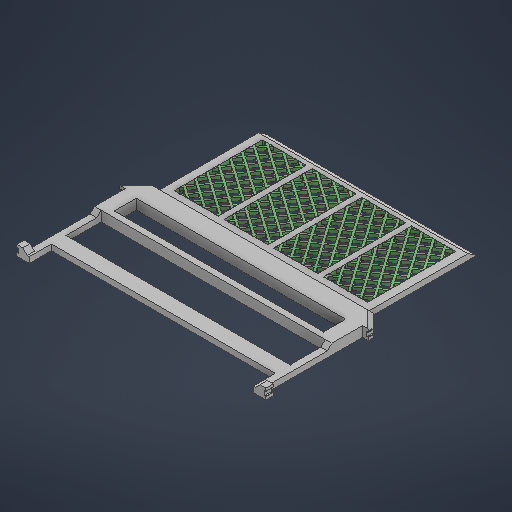
# Autodesk Inventor part: SACMI PH1500 FILLER BOX GRID-DRIVING
Saved by Autodesk Inventor 2025 (Build 290162000, 162)
## iProperties
Created: 2024-05-03
Part Number: SACMI PH1500 FILLER BOX GRID-DRIVING
Material: Generic
Document SubType Name: Modeling
Designer: zulet
Density: 1 g/cm^3
Appearance: Smooth - Medium Gray
Author: zulet
Autodesk Inventor part; units mm, degrees
(part 1 of 2)
ref_plane "YZ Plane" through (0, 0, 0) normal (1, 0, 0) x (0, 1, 0)
ref_plane "XZ Plane" through (0, 0, 0) normal (0, 1, 0) x (-1, 0, 0)
ref_plane "XY Plane" through (0, 0, 0) normal (0, 0, 1) x (1, 0, 0)
sketch "Sketch1" plane through (0, 0, 0) normal (0, 1, 0) x (-1, 0, 0)
  line L0 (-2029.8955, 1380.0763) -> (2005.9504, 1380.0763) construction
  line L1 (2005.9504, 1380.0763) -> (2005.9504, -2689.5627) construction
  line L2 (2005.9504, -2689.5627) -> (-2029.8955, -2689.5627) construction
  line L3 (-2029.8955, -2689.5627) -> (-2029.8955, 1380.0763) construction
  line L4 (810, 0) -> (765, 0)
  line L5 (715, -840) -> (745, -840)
  line L6 (745, -840) -> (850, -735)
  line L7 (850, -735) -> (850, -700)
  line L8 (850, -700) -> (810, -700)
  line L9 (810, -700) -> (810, 0)
  line L10 (715, -840) -> (715, -1515)
  line L11 (715, -1515) -> (0, -1515)
  line L12 (0, -1515) -> (0, -680)
  line L13 (0, -680) -> (715, -680)
  line L14 (765, -490) -> (0, -490)
  line L15 (0, -490) -> (0, -530)
  line L16 (0, -530) -> (715, -530)
  line L17 (715, -530) -> (715, -680)
  line L18 (765, -490) -> (765, -250)
  line L19 (765, -250) -> (0, -250)
  line L20 (0, -250) -> (0, -150)
  line L21 (0, -150) -> (765, -150)
  line L22 (765, -150) -> (765, 0)
  line L23 (810, 0) -> (850, 0)
  line L24 (850, 0) -> (850, -50)
  line L25 (850, -50) -> (810, -50)
  line L26 (810, -50) -> (810, 0)
  line L27 (0, 0) -> (0, -1515) construction
  line L28 (0, 0) -> (850, 0) construction
  line L29 (715, -840) -> (715, -680)
  line L30 (765, -490) -> (810, -490)
  line L31 (715, -840) -> (0, -840)
  point P0 (830, -50)
  point P1 (715, -605)
  point P2 (0, -840)
  dimension "d1" = 4035.8459
  dimension "d24" = 45
  dimension "d25" = 150
  dimension "d26" = 100
  dimension "d27" = 240
  dimension "d28" = 40
  dimension "d29" = 150
  dimension "d32" = 810
  dimension "d33" = 50
  dimension "d43" = 650
  dimension "d45" = 140
  dimension "d46" = 45
  dimension "d48" = 35
  dimension "d49" = 40
  dimension "d50" = 95
  dimension "d57" = 780
  constraints: 56 end point, 13 perpendicular, 7 horizontal, 6 collinear, 4 point on line, 3 vertical, 2 midpoint, 2 parallel, 2 other
  measures "d1" distance of L1.end L2.end
  measures "d24" distance between parallel lines of L22 L9
  measures "d25" distance between parallel lines of L4 L21
  measures "d26" distance between parallel lines of L19 L21
  measures "d27" distance between parallel lines of L14 L19
  measures "d28" distance between parallel lines of L16 L14
  measures "d29" distance between parallel lines of L13 L16
  measures "d32" distance between parallel lines of L27 L9
  measures "d33" distance of L23.end L24.end
  measures "d43" distance from line of point (830, -50) L8
  measures "d45" distance between parallel lines of L8 L5
  measures "d46" angle of L5 L6
  measures "d48" distance of L6.end L7.end
  measures "d49" distance between parallel lines of L9 L24
  measures "d50" distance from line of L9 point (715, -605)
  measures "d57" distance from line of L11 L6.end
extrude "Extrusion1" add sketch "Sketch1" along normal blind 70 contours L23 L24 L25 L9 | L9 L8 L7 L6 L5 L29 L17 L16 L15 L14 L30 | L31 L12 L13 L29
extrude "Extrusion3" add sketch "Sketch1" along normal blind 40 contours L9 L30 L18 L19 L20 L21 L22 L4 | L31 L12 L13 L29 | L10 L11 L12 L31
sketch "Sketch2" plane through (0, 40, 0) normal (0, 1, 0) x (1, 0, 0)
  line L0 (-660, 1485) -> (-360, 1485)
  line L1 (-360, 1485) -> (-360, 885)
  line L2 (-360, 885) -> (-660, 885)
  line L3 (-660, 885) -> (-660, 1485)
  line L4 (0, 1515) -> (-715, 1515) projected
  line L5 (-850, 735) -> (-850, 700) projected
  line L6 (-320, 885) -> (-20, 885)
  line L7 (-20, 885) -> (-20, 1485)
  line L8 (-20, 1485) -> (-320, 1485)
  line L9 (-320, 1485) -> (-320, 885)
  point P0 (0, 0)
  dimension "d58" = 300
  dimension "d59" = 600
  dimension "d60" = 30
  dimension "d61" = 190
  dimension "d62" = 300
  dimension "d63" = 600
  dimension "d64" = 40
  dimension "d65" = 30
  constraints: 16 end point, 4 parallel, 2 horizontal, 2 perpendicular
  measures "d58" distance of L1.end L2.end
  measures "d59" distance of L0.end L1.end
  measures "d60" distance between parallel lines of L4 L0
  measures "d61" distance between parallel lines of L3 L5
  measures "d62" distance of L8.end L7.end
  measures "d63" distance of L7.end L6.end
  measures "d64" distance between parallel lines of L1 L9
  measures "d65" distance between parallel lines of L4 L8
extrude "Extrusion4" cut sketch "Sketch2" against normal blind 40
sketch "Sketch3" plane through (0, 40, 0) normal (0, 1, 0) x (1, 0, 0)
  line L0 (273.75, 1258.6647) -> (232.7924, 1287.3435)
  line L1 (232.7924, 1287.3435) -> (261.4712, 1328.3011)
  line L2 (261.4712, 1328.3011) -> (302.4288, 1299.6223)
  line L3 (302.4288, 1299.6223) -> (273.75, 1258.6647)
  line L4 (-360, 885) -> (-660, 885) projected
  line L5 (220.5051, 1295.9471) -> (179.5475, 1324.626)
  line L6 (179.5475, 1324.626) -> (208.2263, 1365.5836)
  line L7 (208.2263, 1365.5836) -> (249.1839, 1336.9047)
  line L8 (249.1839, 1336.9047) -> (220.5051, 1295.9471)
  line L9 (167.2602, 1333.2296) -> (126.3026, 1361.9084)
  line L10 (126.3026, 1361.9084) -> (154.9815, 1402.866)
  line L11 (154.9815, 1402.866) -> (195.9391, 1374.1872)
  line L12 (195.9391, 1374.1872) -> (167.2602, 1333.2296)
  line L13 (114.0154, 1370.5121) -> (73.0577, 1399.1909)
  line L14 (73.0577, 1399.1909) -> (101.7366, 1440.1485)
  line L15 (101.7366, 1440.1485) -> (142.6942, 1411.4697)
  line L16 (142.6942, 1411.4697) -> (114.0154, 1370.5121)
  line L17 (60.7705, 1407.7945) -> (19.8129, 1436.4734)
  line L18 (19.8129, 1436.4734) -> (48.4917, 1477.431)
  line L19 (48.4917, 1477.431) -> (89.4493, 1448.7521)
  line L20 (89.4493, 1448.7521) -> (60.7705, 1407.7945)
  line L21 (7.5256, 1445.077) -> (-33.432, 1473.7558)
  line L22 (-33.432, 1473.7558) -> (-4.7532, 1514.7134)
  line L23 (-4.7532, 1514.7134) -> (36.2044, 1486.0346)
  line L24 (36.2044, 1486.0346) -> (7.5256, 1445.077)
  line L25 (-45.7193, 1482.3595) -> (-86.6769, 1511.0383)
  line L26 (-86.6769, 1511.0383) -> (-57.9981, 1551.9959)
  line L27 (-57.9981, 1551.9959) -> (-17.0405, 1523.3171)
  line L28 (-17.0405, 1523.3171) -> (-45.7193, 1482.3595)
  line L29 (-98.9642, 1519.6419) -> (-139.9218, 1548.3208)
  line L30 (-139.9218, 1548.3208) -> (-111.243, 1589.2784)
  line L31 (-111.243, 1589.2784) -> (-70.2854, 1560.5995)
  line L32 (-70.2854, 1560.5995) -> (-98.9642, 1519.6419)
  line L33 (-152.2091, 1556.9244) -> (-193.1667, 1585.6032)
  line L34 (-193.1667, 1585.6032) -> (-164.4878, 1626.5608)
  line L35 (-164.4878, 1626.5608) -> (-123.5302, 1597.882)
  line L36 (-123.5302, 1597.882) -> (-152.2091, 1556.9244)
  line L37 (-205.4539, 1594.2069) -> (-246.4115, 1622.8857)
  line L38 (-246.4115, 1622.8857) -> (-217.7327, 1663.8433)
  line L39 (-217.7327, 1663.8433) -> (-176.7751, 1635.1645)
  line L40 (-176.7751, 1635.1645) -> (-205.4539, 1594.2069)
  line L41 (-258.6988, 1631.4894) -> (-299.6564, 1660.1682)
  line L42 (-299.6564, 1660.1682) -> (-270.9776, 1701.1258)
  line L43 (-270.9776, 1701.1258) -> (-230.02, 1672.447)
  line L44 (-230.02, 1672.447) -> (-258.6988, 1631.4894)
  line L45 (-311.9437, 1668.7718) -> (-352.9013, 1697.4506)
  line L46 (-352.9013, 1697.4506) -> (-324.2225, 1738.4082)
  line L47 (-324.2225, 1738.4082) -> (-283.2649, 1709.7294)
  line L48 (-283.2649, 1709.7294) -> (-311.9437, 1668.7718)
  line L49 (-365.1886, 1706.0543) -> (-406.1462, 1734.7331)
  line L50 (-406.1462, 1734.7331) -> (-377.4674, 1775.6907)
  line L51 (-377.4674, 1775.6907) -> (-336.5098, 1747.0119)
  line L52 (-336.5098, 1747.0119) -> (-365.1886, 1706.0543)
  line L53 (-418.4335, 1743.3368) -> (-459.3911, 1772.0156)
  line L54 (-459.3911, 1772.0156) -> (-430.7123, 1812.9732)
  line L55 (-430.7123, 1812.9732) -> (-389.7547, 1784.2944)
  line L56 (-389.7547, 1784.2944) -> (-418.4335, 1743.3368)
  line L57 (-471.6784, 1780.6192) -> (-512.636, 1809.298)
  line L58 (-512.636, 1809.298) -> (-483.9571, 1850.2556)
  line L59 (-483.9571, 1850.2556) -> (-442.9995, 1821.5768)
  line L60 (-442.9995, 1821.5768) -> (-471.6784, 1780.6192)
  line L61 (236.4675, 1205.4198) -> (195.5099, 1234.0986)
  line L62 (195.5099, 1234.0986) -> (224.1888, 1275.0562)
  line L63 (224.1888, 1275.0562) -> (265.1464, 1246.3774)
  line L64 (265.1464, 1246.3774) -> (236.4675, 1205.4198)
  line L65 (183.2226, 1242.7023) -> (142.265, 1271.3811)
  line L66 (142.265, 1271.3811) -> (170.9439, 1312.3387)
  line L67 (170.9439, 1312.3387) -> (211.9015, 1283.6599)
  line L68 (211.9015, 1283.6599) -> (183.2226, 1242.7023)
  line L69 (129.9778, 1279.9847) -> (89.0202, 1308.6635)
  line L70 (89.0202, 1308.6635) -> (117.699, 1349.6211)
  line L71 (117.699, 1349.6211) -> (158.6566, 1320.9423)
  line L72 (158.6566, 1320.9423) -> (129.9778, 1279.9847)
  line L73 (76.7329, 1317.2672) -> (35.7753, 1345.946)
  line L74 (35.7753, 1345.946) -> (64.4541, 1386.9036)
  line L75 (64.4541, 1386.9036) -> (105.4117, 1358.2248)
  line L76 (105.4117, 1358.2248) -> (76.7329, 1317.2672)
  line L77 (23.488, 1354.5497) -> (-17.4696, 1383.2285)
  line L78 (-17.4696, 1383.2285) -> (11.2092, 1424.1861)
  line L79 (11.2092, 1424.1861) -> (52.1668, 1395.5073)
  line L80 (52.1668, 1395.5073) -> (23.488, 1354.5497)
  line L81 (-29.7569, 1391.8321) -> (-70.7145, 1420.5109)
  line L82 (-70.7145, 1420.5109) -> (-42.0357, 1461.4686)
  line L83 (-42.0357, 1461.4686) -> (-1.0781, 1432.7897)
  line L84 (-1.0781, 1432.7897) -> (-29.7569, 1391.8321)
  line L85 (-83.0018, 1429.1146) -> (-123.9594, 1457.7934)
  line L86 (-123.9594, 1457.7934) -> (-95.2805, 1498.751)
  line L87 (-95.2805, 1498.751) -> (-54.3229, 1470.0722)
  line L88 (-54.3229, 1470.0722) -> (-83.0018, 1429.1146)
  line L89 (-136.2466, 1466.3971) -> (-177.2043, 1495.0759)
  line L90 (-177.2043, 1495.0759) -> (-148.5254, 1536.0335)
  line L91 (-148.5254, 1536.0335) -> (-107.5678, 1507.3547)
  line L92 (-107.5678, 1507.3547) -> (-136.2466, 1466.3971)
  line L93 (-189.4915, 1503.6795) -> (-230.4491, 1532.3584)
  line L94 (-230.4491, 1532.3584) -> (-201.7703, 1573.316)
  line L95 (-201.7703, 1573.316) -> (-160.8127, 1544.6371)
  line L96 (-160.8127, 1544.6371) -> (-189.4915, 1503.6795)
  line L97 (-242.7364, 1540.962) -> (-283.694, 1569.6408)
  line L98 (-283.694, 1569.6408) -> (-255.0152, 1610.5984)
  line L99 (-255.0152, 1610.5984) -> (-214.0576, 1581.9196)
  line L100 (-214.0576, 1581.9196) -> (-242.7364, 1540.962)
  line L101 (-295.9813, 1578.2445) -> (-336.9389, 1606.9233)
  line L102 (-336.9389, 1606.9233) -> (-308.2601, 1647.8809)
  line L103 (-308.2601, 1647.8809) -> (-267.3025, 1619.2021)
  line L104 (-267.3025, 1619.2021) -> (-295.9813, 1578.2445)
  line L105 (-349.2262, 1615.5269) -> (-390.1838, 1644.2058)
  line L106 (-390.1838, 1644.2058) -> (-361.505, 1685.1634)
  line L107 (-361.505, 1685.1634) -> (-320.5474, 1656.4845)
  line L108 (-320.5474, 1656.4845) -> (-349.2262, 1615.5269)
  line L109 (-402.4711, 1652.8094) -> (-443.4287, 1681.4882)
  line L110 (-443.4287, 1681.4882) -> (-414.7498, 1722.4458)
  line L111 (-414.7498, 1722.4458) -> (-373.7922, 1693.767)
  line L112 (-373.7922, 1693.767) -> (-402.4711, 1652.8094)
  line L113 (-455.7159, 1690.0919) -> (-496.6735, 1718.7707)
  line L114 (-496.6735, 1718.7707) -> (-467.9947, 1759.7283)
  line L115 (-467.9947, 1759.7283) -> (-427.0371, 1731.0495)
  line L116 (-427.0371, 1731.0495) -> (-455.7159, 1690.0919)
  line L117 (-508.9608, 1727.3743) -> (-549.9184, 1756.0532)
  line L118 (-549.9184, 1756.0532) -> (-521.2396, 1797.0108)
  line L119 (-521.2396, 1797.0108) -> (-480.282, 1768.3319)
  line L120 (-480.282, 1768.3319) -> (-508.9608, 1727.3743)
  line L121 (199.1851, 1152.1749) -> (158.2275, 1180.8537)
  line L122 (158.2275, 1180.8537) -> (186.9063, 1221.8113)
  line L123 (186.9063, 1221.8113) -> (227.8639, 1193.1325)
  line L124 (227.8639, 1193.1325) -> (199.1851, 1152.1749)
  line L125 (145.9402, 1189.4574) -> (104.9826, 1218.1362)
  line L126 (104.9826, 1218.1362) -> (133.6614, 1259.0938)
  line L127 (133.6614, 1259.0938) -> (174.619, 1230.415)
  line L128 (174.619, 1230.415) -> (145.9402, 1189.4574)
  line L129 (92.6953, 1226.7398) -> (51.7377, 1255.4187)
  line L130 (51.7377, 1255.4187) -> (80.4165, 1296.3763)
  line L131 (80.4165, 1296.3763) -> (121.3741, 1267.6974)
  line L132 (121.3741, 1267.6974) -> (92.6953, 1226.7398)
  line L133 (39.4504, 1264.0223) -> (-1.5072, 1292.7011)
  line L134 (-1.5072, 1292.7011) -> (27.1716, 1333.6587)
  line L135 (27.1716, 1333.6587) -> (68.1292, 1304.9799)
  line L136 (68.1292, 1304.9799) -> (39.4504, 1264.0223)
  line L137 (-13.7945, 1301.3048) -> (-54.7521, 1329.9836)
  line L138 (-54.7521, 1329.9836) -> (-26.0732, 1370.9412)
  line L139 (-26.0732, 1370.9412) -> (14.8844, 1342.2624)
  line L140 (14.8844, 1342.2624) -> (-13.7945, 1301.3048)
  line L141 (-67.0394, 1338.5872) -> (-107.997, 1367.2661)
  line L142 (-107.997, 1367.2661) -> (-79.3181, 1408.2237)
  line L143 (-79.3181, 1408.2237) -> (-38.3605, 1379.5448)
  line L144 (-38.3605, 1379.5448) -> (-67.0394, 1338.5872)
  line L145 (-120.2842, 1375.8697) -> (-161.2418, 1404.5485)
  line L146 (-161.2418, 1404.5485) -> (-132.563, 1445.5061)
  line L147 (-132.563, 1445.5061) -> (-91.6054, 1416.8273)
  line L148 (-91.6054, 1416.8273) -> (-120.2842, 1375.8697)
  line L149 (-173.5291, 1413.1522) -> (-214.4867, 1441.831)
  line L150 (-214.4867, 1441.831) -> (-185.8079, 1482.7886)
  line L151 (-185.8079, 1482.7886) -> (-144.8503, 1454.1098)
  line L152 (-144.8503, 1454.1098) -> (-173.5291, 1413.1522)
  line L153 (-226.774, 1450.4346) -> (-267.7316, 1479.1135)
  line L154 (-267.7316, 1479.1135) -> (-239.0528, 1520.0711)
  line L155 (-239.0528, 1520.0711) -> (-198.0952, 1491.3923)
  line L156 (-198.0952, 1491.3923) -> (-226.774, 1450.4346)
  line L157 (-280.0189, 1487.7171) -> (-320.9765, 1516.3959)
  line L158 (-320.9765, 1516.3959) -> (-292.2977, 1557.3535)
  line L159 (-292.2977, 1557.3535) -> (-251.3401, 1528.6747)
  line L160 (-251.3401, 1528.6747) -> (-280.0189, 1487.7171)
  line L161 (-333.2638, 1524.9996) -> (-374.2214, 1553.6784)
  line L162 (-374.2214, 1553.6784) -> (-345.5425, 1594.636)
  line L163 (-345.5425, 1594.636) -> (-304.5849, 1565.9572)
  line L164 (-304.5849, 1565.9572) -> (-333.2638, 1524.9996)
  line L165 (-386.5086, 1562.2821) -> (-427.4663, 1590.9609)
  line L166 (-427.4663, 1590.9609) -> (-398.7874, 1631.9185)
  line L167 (-398.7874, 1631.9185) -> (-357.8298, 1603.2397)
  line L168 (-357.8298, 1603.2397) -> (-386.5086, 1562.2821)
  line L169 (-439.7535, 1599.5645) -> (-480.7111, 1628.2433)
  line L170 (-480.7111, 1628.2433) -> (-452.0323, 1669.2009)
  line L171 (-452.0323, 1669.2009) -> (-411.0747, 1640.5221)
  line L172 (-411.0747, 1640.5221) -> (-439.7535, 1599.5645)
  line L173 (-492.9984, 1636.847) -> (-533.956, 1665.5258)
  line L174 (-533.956, 1665.5258) -> (-505.2772, 1706.4834)
  line L175 (-505.2772, 1706.4834) -> (-464.3196, 1677.8046)
  line L176 (-464.3196, 1677.8046) -> (-492.9984, 1636.847)
  line L177 (-546.2433, 1674.1295) -> (-587.2009, 1702.8083)
  line L178 (-587.2009, 1702.8083) -> (-558.5221, 1743.7659)
  line L179 (-558.5221, 1743.7659) -> (-517.5645, 1715.0871)
  line L180 (-517.5645, 1715.0871) -> (-546.2433, 1674.1295)
  line L181 (161.9026, 1098.93) -> (120.945, 1127.6088)
  line L182 (120.945, 1127.6088) -> (149.6238, 1168.5664)
  line L183 (149.6238, 1168.5664) -> (190.5814, 1139.8876)
  line L184 (190.5814, 1139.8876) -> (161.9026, 1098.93)
  line L185 (108.6577, 1136.2125) -> (67.7001, 1164.8913)
  line L186 (67.7001, 1164.8913) -> (96.3789, 1205.8489)
  line L187 (96.3789, 1205.8489) -> (137.3365, 1177.1701)
  line L188 (137.3365, 1177.1701) -> (108.6577, 1136.2125)
  line L189 (55.4128, 1173.495) -> (14.4552, 1202.1738)
  line L190 (14.4552, 1202.1738) -> (43.134, 1243.1314)
  line L191 (43.134, 1243.1314) -> (84.0917, 1214.4526)
  line L192 (84.0917, 1214.4526) -> (55.4128, 1173.495)
  line L193 (2.1679, 1210.7774) -> (-38.7897, 1239.4562)
  line L194 (-38.7897, 1239.4562) -> (-10.1108, 1280.4138)
  line L195 (-10.1108, 1280.4138) -> (30.8468, 1251.735)
  line L196 (30.8468, 1251.735) -> (2.1679, 1210.7774)
  line L197 (-51.0769, 1248.0599) -> (-92.0345, 1276.7387)
  line L198 (-92.0345, 1276.7387) -> (-63.3557, 1317.6963)
  line L199 (-63.3557, 1317.6963) -> (-22.3981, 1289.0175)
  line L200 (-22.3981, 1289.0175) -> (-51.0769, 1248.0599)
  line L201 (-104.3218, 1285.3424) -> (-145.2794, 1314.0212)
  line L202 (-145.2794, 1314.0212) -> (-116.6006, 1354.9788)
  line L203 (-116.6006, 1354.9788) -> (-75.643, 1326.3)
  line L204 (-75.643, 1326.3) -> (-104.3218, 1285.3424)
  line L205 (-157.5667, 1322.6248) -> (-198.5243, 1351.3037)
  line L206 (-198.5243, 1351.3037) -> (-169.8455, 1392.2613)
  line L207 (-169.8455, 1392.2613) -> (-128.8879, 1363.5824)
  line L208 (-128.8879, 1363.5824) -> (-157.5667, 1322.6248)
  line L209 (-210.8116, 1359.9073) -> (-251.7692, 1388.5861)
  line L210 (-251.7692, 1388.5861) -> (-223.0904, 1429.5437)
  line L211 (-223.0904, 1429.5437) -> (-182.1328, 1400.8649)
  line L212 (-182.1328, 1400.8649) -> (-210.8116, 1359.9073)
  line L213 (-264.0565, 1397.1898) -> (-305.0141, 1425.8686)
  line L214 (-305.0141, 1425.8686) -> (-276.3352, 1466.8262)
  line L215 (-276.3352, 1466.8262) -> (-235.3776, 1438.1474)
  line L216 (-235.3776, 1438.1474) -> (-264.0565, 1397.1898)
  line L217 (-317.3014, 1434.4722) -> (-358.259, 1463.1511)
  line L218 (-358.259, 1463.1511) -> (-329.5801, 1504.1087)
  line L219 (-329.5801, 1504.1087) -> (-288.6225, 1475.4298)
  line L220 (-288.6225, 1475.4298) -> (-317.3014, 1434.4722)
  line L221 (-370.5462, 1471.7547) -> (-411.5038, 1500.4335)
  line L222 (-411.5038, 1500.4335) -> (-382.825, 1541.3911)
  line L223 (-382.825, 1541.3911) -> (-341.8674, 1512.7123)
  line L224 (-341.8674, 1512.7123) -> (-370.5462, 1471.7547)
  line L225 (-423.7911, 1509.0372) -> (-464.7487, 1537.716)
  line L226 (-464.7487, 1537.716) -> (-436.0699, 1578.6736)
  line L227 (-436.0699, 1578.6736) -> (-395.1123, 1549.9948)
  line L228 (-395.1123, 1549.9948) -> (-423.7911, 1509.0372)
  line L229 (-477.036, 1546.3196) -> (-517.9936, 1574.9985)
  line L230 (-517.9936, 1574.9985) -> (-489.3148, 1615.9561)
  line L231 (-489.3148, 1615.9561) -> (-448.3572, 1587.2772)
  line L232 (-448.3572, 1587.2772) -> (-477.036, 1546.3196)
  line L233 (-530.2809, 1583.6021) -> (-571.2385, 1612.2809)
  line L234 (-571.2385, 1612.2809) -> (-542.5597, 1653.2385)
  line L235 (-542.5597, 1653.2385) -> (-501.6021, 1624.5597)
  line L236 (-501.6021, 1624.5597) -> (-530.2809, 1583.6021)
  line L237 (-583.5258, 1620.8846) -> (-624.4834, 1649.5634)
  line L238 (-624.4834, 1649.5634) -> (-595.8045, 1690.521)
  line L239 (-595.8045, 1690.521) -> (-554.8469, 1661.8422)
  line L240 (-554.8469, 1661.8422) -> (-583.5258, 1620.8846)
  line L241 (124.6201, 1045.6851) -> (83.6625, 1074.364)
  line L242 (83.6625, 1074.364) -> (112.3413, 1115.3216)
  line L243 (112.3413, 1115.3216) -> (153.2989, 1086.6427)
  line L244 (153.2989, 1086.6427) -> (124.6201, 1045.6851)
  line L245 (71.3752, 1082.9676) -> (30.4176, 1111.6464)
  line L246 (30.4176, 1111.6464) -> (59.0965, 1152.604)
  line L247 (59.0965, 1152.604) -> (100.0541, 1123.9252)
  line L248 (100.0541, 1123.9252) -> (71.3752, 1082.9676)
  line L249 (18.1304, 1120.2501) -> (-22.8272, 1148.9289)
  line L250 (-22.8272, 1148.9289) -> (5.8516, 1189.8865)
  line L251 (5.8516, 1189.8865) -> (46.8092, 1161.2077)
  line L252 (46.8092, 1161.2077) -> (18.1304, 1120.2501)
  line L253 (-35.1145, 1157.5325) -> (-76.0721, 1186.2114)
  line L254 (-76.0721, 1186.2114) -> (-47.3933, 1227.169)
  line L255 (-47.3933, 1227.169) -> (-6.4357, 1198.4901)
  line L256 (-6.4357, 1198.4901) -> (-35.1145, 1157.5325)
  line L257 (-88.3594, 1194.815) -> (-129.317, 1223.4938)
  line L258 (-129.317, 1223.4938) -> (-100.6382, 1264.4514)
  line L259 (-100.6382, 1264.4514) -> (-59.6806, 1235.7726)
  line L260 (-59.6806, 1235.7726) -> (-88.3594, 1194.815)
  line L261 (-141.6043, 1232.0975) -> (-182.5619, 1260.7763)
  line L262 (-182.5619, 1260.7763) -> (-153.8831, 1301.7339)
  line L263 (-153.8831, 1301.7339) -> (-112.9255, 1273.0551)
  line L264 (-112.9255, 1273.0551) -> (-141.6043, 1232.0975)
  line L265 (-194.8492, 1269.3799) -> (-235.8068, 1298.0588)
  line L266 (-235.8068, 1298.0588) -> (-207.128, 1339.0164)
  line L267 (-207.128, 1339.0164) -> (-166.1703, 1310.3375)
  line L268 (-166.1703, 1310.3375) -> (-194.8492, 1269.3799)
  line L269 (-248.0941, 1306.6624) -> (-289.0517, 1335.3412)
  line L270 (-289.0517, 1335.3412) -> (-260.3728, 1376.2988)
  line L271 (-260.3728, 1376.2988) -> (-219.4152, 1347.62)
  line L272 (-219.4152, 1347.62) -> (-248.0941, 1306.6624)
  line L273 (-301.3389, 1343.9449) -> (-342.2965, 1372.6237)
  line L274 (-342.2965, 1372.6237) -> (-313.6177, 1413.5813)
  line L275 (-313.6177, 1413.5813) -> (-272.6601, 1384.9025)
  line L276 (-272.6601, 1384.9025) -> (-301.3389, 1343.9449)
  line L277 (-354.5838, 1381.2274) -> (-395.5414, 1409.9062)
  line L278 (-395.5414, 1409.9062) -> (-366.8626, 1450.8638)
  line L279 (-366.8626, 1450.8638) -> (-325.905, 1422.185)
  line L280 (-325.905, 1422.185) -> (-354.5838, 1381.2274)
  line L281 (-407.8287, 1418.5098) -> (-448.7863, 1447.1886)
  line L282 (-448.7863, 1447.1886) -> (-420.1075, 1488.1462)
  line L283 (-420.1075, 1488.1462) -> (-379.1499, 1459.4674)
  line L284 (-379.1499, 1459.4674) -> (-407.8287, 1418.5098)
  line L285 (-461.0736, 1455.7923) -> (-502.0312, 1484.4711)
  line L286 (-502.0312, 1484.4711) -> (-473.3524, 1525.4287)
  line L287 (-473.3524, 1525.4287) -> (-432.3948, 1496.7499)
  line L288 (-432.3948, 1496.7499) -> (-461.0736, 1455.7923)
  line L289 (-514.3185, 1493.0748) -> (-555.2761, 1521.7536)
  line L290 (-555.2761, 1521.7536) -> (-526.5972, 1562.7112)
  line L291 (-526.5972, 1562.7112) -> (-485.6396, 1534.0324)
  line L292 (-485.6396, 1534.0324) -> (-514.3185, 1493.0748)
  line L293 (-567.5634, 1530.3572) -> (-608.521, 1559.036)
  line L294 (-608.521, 1559.036) -> (-579.8421, 1599.9936)
  line L295 (-579.8421, 1599.9936) -> (-538.8845, 1571.3148)
  line L296 (-538.8845, 1571.3148) -> (-567.5634, 1530.3572)
  line L297 (-620.8082, 1567.6397) -> (-661.7658, 1596.3185)
  line L298 (-661.7658, 1596.3185) -> (-633.087, 1637.2761)
  line L299 (-633.087, 1637.2761) -> (-592.1294, 1608.5973)
  line L300 (-592.1294, 1608.5973) -> (-620.8082, 1567.6397)
  line L301 (87.3377, 992.4403) -> (46.3801, 1021.1191)
  line L302 (46.3801, 1021.1191) -> (75.0589, 1062.0767)
  line L303 (75.0589, 1062.0767) -> (116.0165, 1033.3979)
  line L304 (116.0165, 1033.3979) -> (87.3377, 992.4403)
  line L305 (34.0928, 1029.7227) -> (-6.8648, 1058.4015)
  line L306 (-6.8648, 1058.4015) -> (21.814, 1099.3591)
  line L307 (21.814, 1099.3591) -> (62.7716, 1070.6803)
  line L308 (62.7716, 1070.6803) -> (34.0928, 1029.7227)
  line L309 (-19.1521, 1067.0052) -> (-60.1097, 1095.684)
  line L310 (-60.1097, 1095.684) -> (-31.4309, 1136.6416)
  line L311 (-31.4309, 1136.6416) -> (9.5267, 1107.9628)
  line L312 (9.5267, 1107.9628) -> (-19.1521, 1067.0052)
  line L313 (-72.397, 1104.2877) -> (-113.3546, 1132.9665)
  line L314 (-113.3546, 1132.9665) -> (-84.6758, 1173.9241)
  line L315 (-84.6758, 1173.9241) -> (-43.7182, 1145.2453)
  line L316 (-43.7182, 1145.2453) -> (-72.397, 1104.2877)
  line L317 (-125.6419, 1141.5701) -> (-166.5995, 1170.2489)
  line L318 (-166.5995, 1170.2489) -> (-137.9207, 1211.2066)
  line L319 (-137.9207, 1211.2066) -> (-96.9631, 1182.5277)
  line L320 (-96.9631, 1182.5277) -> (-125.6419, 1141.5701)
  line L321 (-178.8868, 1178.8526) -> (-219.8444, 1207.5314)
  line L322 (-219.8444, 1207.5314) -> (-191.1655, 1248.489)
  line L323 (-191.1655, 1248.489) -> (-150.2079, 1219.8102)
  line L324 (-150.2079, 1219.8102) -> (-178.8868, 1178.8526)
  line L325 (-232.1316, 1216.1351) -> (-273.0892, 1244.8139)
  line L326 (-273.0892, 1244.8139) -> (-244.4104, 1285.7715)
  line L327 (-244.4104, 1285.7715) -> (-203.4528, 1257.0927)
  line L328 (-203.4528, 1257.0927) -> (-232.1316, 1216.1351)
  line L329 (-285.3765, 1253.4175) -> (-326.3341, 1282.0964)
  line L330 (-326.3341, 1282.0964) -> (-297.6553, 1323.054)
  line L331 (-297.6553, 1323.054) -> (-256.6977, 1294.3751)
  line L332 (-256.6977, 1294.3751) -> (-285.3765, 1253.4175)
  line L333 (-338.6214, 1290.7) -> (-379.579, 1319.3788)
  line L334 (-379.579, 1319.3788) -> (-350.9002, 1360.3364)
  line L335 (-350.9002, 1360.3364) -> (-309.9426, 1331.6576)
  line L336 (-309.9426, 1331.6576) -> (-338.6214, 1290.7)
  line L337 (-391.8663, 1327.9825) -> (-432.8239, 1356.6613)
  line L338 (-432.8239, 1356.6613) -> (-404.1451, 1397.6189)
  line L339 (-404.1451, 1397.6189) -> (-363.1875, 1368.9401)
  line L340 (-363.1875, 1368.9401) -> (-391.8663, 1327.9825)
  line L341 (-445.1112, 1365.2649) -> (-486.0688, 1393.9438)
  line L342 (-486.0688, 1393.9438) -> (-457.39, 1434.9014)
  line L343 (-457.39, 1434.9014) -> (-416.4323, 1406.2225)
  line L344 (-416.4323, 1406.2225) -> (-445.1112, 1365.2649)
  line L345 (-498.3561, 1402.5474) -> (-539.3137, 1431.2262)
  line L346 (-539.3137, 1431.2262) -> (-510.6348, 1472.1838)
  line L347 (-510.6348, 1472.1838) -> (-469.6772, 1443.505)
  line L348 (-469.6772, 1443.505) -> (-498.3561, 1402.5474)
  line L349 (-551.6009, 1439.8299) -> (-592.5585, 1468.5087)
  line L350 (-592.5585, 1468.5087) -> (-563.8797, 1509.4663)
  line L351 (-563.8797, 1509.4663) -> (-522.9221, 1480.7875)
  line L352 (-522.9221, 1480.7875) -> (-551.6009, 1439.8299)
  line L353 (-604.8458, 1477.1123) -> (-645.8034, 1505.7912)
  line L354 (-645.8034, 1505.7912) -> (-617.1246, 1546.7488)
  line L355 (-617.1246, 1546.7488) -> (-576.167, 1518.0699)
  line L356 (-576.167, 1518.0699) -> (-604.8458, 1477.1123)
  line L357 (-658.0907, 1514.3948) -> (-699.0483, 1543.0736)
  line L358 (-699.0483, 1543.0736) -> (-670.3695, 1584.0312)
  line L359 (-670.3695, 1584.0312) -> (-629.4119, 1555.3524)
  line L360 (-629.4119, 1555.3524) -> (-658.0907, 1514.3948)
  line L361 (50.0552, 939.1954) -> (9.0976, 967.8742)
  line L362 (9.0976, 967.8742) -> (37.7764, 1008.8318)
  line L363 (37.7764, 1008.8318) -> (78.734, 980.153)
  line L364 (78.734, 980.153) -> (50.0552, 939.1954)
  line L365 (-3.1897, 976.4778) -> (-44.1473, 1005.1567)
  line L366 (-44.1473, 1005.1567) -> (-15.4685, 1046.1143)
  line L367 (-15.4685, 1046.1143) -> (25.4891, 1017.4354)
  line L368 (25.4891, 1017.4354) -> (-3.1897, 976.4778)
  line L369 (-56.4346, 1013.7603) -> (-97.3922, 1042.4391)
  line L370 (-97.3922, 1042.4391) -> (-68.7134, 1083.3967)
  line L371 (-68.7134, 1083.3967) -> (-27.7558, 1054.7179)
  line L372 (-27.7558, 1054.7179) -> (-56.4346, 1013.7603)
  line L373 (-109.6795, 1051.0428) -> (-150.6371, 1079.7216)
  line L374 (-150.6371, 1079.7216) -> (-121.9582, 1120.6792)
  line L375 (-121.9582, 1120.6792) -> (-81.0006, 1092.0004)
  line L376 (-81.0006, 1092.0004) -> (-109.6795, 1051.0428)
  line L377 (-162.9243, 1088.3252) -> (-203.8819, 1117.0041)
  line L378 (-203.8819, 1117.0041) -> (-175.2031, 1157.9617)
  line L379 (-175.2031, 1157.9617) -> (-134.2455, 1129.2828)
  line L380 (-134.2455, 1129.2828) -> (-162.9243, 1088.3252)
  line L381 (-216.1692, 1125.6077) -> (-257.1268, 1154.2865)
  line L382 (-257.1268, 1154.2865) -> (-228.448, 1195.2441)
  line L383 (-228.448, 1195.2441) -> (-187.4904, 1166.5653)
  line L384 (-187.4904, 1166.5653) -> (-216.1692, 1125.6077)
  line L385 (-269.4141, 1162.8902) -> (-310.3717, 1191.569)
  line L386 (-310.3717, 1191.569) -> (-281.6929, 1232.5266)
  line L387 (-281.6929, 1232.5266) -> (-240.7353, 1203.8478)
  line L388 (-240.7353, 1203.8478) -> (-269.4141, 1162.8902)
  line L389 (-322.659, 1200.1726) -> (-363.6166, 1228.8515)
  line L390 (-363.6166, 1228.8515) -> (-334.9378, 1269.8091)
  line L391 (-334.9378, 1269.8091) -> (-293.9802, 1241.1303)
  line L392 (-293.9802, 1241.1303) -> (-322.659, 1200.1726)
  line L393 (-375.9039, 1237.4551) -> (-416.8615, 1266.1339)
  line L394 (-416.8615, 1266.1339) -> (-388.1827, 1307.0915)
  line L395 (-388.1827, 1307.0915) -> (-347.2251, 1278.4127)
  line L396 (-347.2251, 1278.4127) -> (-375.9039, 1237.4551)
  line L397 (-429.1488, 1274.7376) -> (-470.1064, 1303.4164)
  line L398 (-470.1064, 1303.4164) -> (-441.4275, 1344.374)
  line L399 (-441.4275, 1344.374) -> (-400.4699, 1315.6952)
  line L400 (-400.4699, 1315.6952) -> (-429.1488, 1274.7376)
  line L401 (-482.3936, 1312.0201) -> (-523.3512, 1340.6989)
  line L402 (-523.3512, 1340.6989) -> (-494.6724, 1381.6565)
  line L403 (-494.6724, 1381.6565) -> (-453.7148, 1352.9777)
  line L404 (-453.7148, 1352.9777) -> (-482.3936, 1312.0201)
  line L405 (-535.6385, 1349.3025) -> (-576.5961, 1377.9813)
  line L406 (-576.5961, 1377.9813) -> (-547.9173, 1418.9389)
  line L407 (-547.9173, 1418.9389) -> (-506.9597, 1390.2601)
  line L408 (-506.9597, 1390.2601) -> (-535.6385, 1349.3025)
  line L409 (-588.8834, 1386.585) -> (-629.841, 1415.2638)
  line L410 (-629.841, 1415.2638) -> (-601.1622, 1456.2214)
  line L411 (-601.1622, 1456.2214) -> (-560.2046, 1427.5426)
  line L412 (-560.2046, 1427.5426) -> (-588.8834, 1386.585)
  line L413 (-642.1283, 1423.8675) -> (-683.0859, 1452.5463)
  line L414 (-683.0859, 1452.5463) -> (-654.4071, 1493.5039)
  line L415 (-654.4071, 1493.5039) -> (-613.4495, 1464.8251)
  line L416 (-613.4495, 1464.8251) -> (-642.1283, 1423.8675)
  line L417 (-695.3732, 1461.1499) -> (-736.3308, 1489.8287)
  line L418 (-736.3308, 1489.8287) -> (-707.652, 1530.7864)
  line L419 (-707.652, 1530.7864) -> (-666.6943, 1502.1075)
  line L420 (-666.6943, 1502.1075) -> (-695.3732, 1461.1499)
  line L421 (12.7727, 885.9505) -> (-28.1849, 914.6293)
  line L422 (-28.1849, 914.6293) -> (0.4939, 955.5869)
  line L423 (0.4939, 955.5869) -> (41.4515, 926.9081)
  line L424 (41.4515, 926.9081) -> (12.7727, 885.9505)
  line L425 (-40.4722, 923.233) -> (-81.4298, 951.9118)
  line L426 (-81.4298, 951.9118) -> (-52.7509, 992.8694)
  line L427 (-52.7509, 992.8694) -> (-11.7933, 964.1906)
  line L428 (-11.7933, 964.1906) -> (-40.4722, 923.233)
  line L429 (-93.717, 960.5154) -> (-134.6746, 989.1942)
  line L430 (-134.6746, 989.1942) -> (-105.9958, 1030.1518)
  line L431 (-105.9958, 1030.1518) -> (-65.0382, 1001.473)
  line L432 (-65.0382, 1001.473) -> (-93.717, 960.5154)
  line L433 (-146.9619, 997.7979) -> (-187.9195, 1026.4767)
  line L434 (-187.9195, 1026.4767) -> (-159.2407, 1067.4343)
  line L435 (-159.2407, 1067.4343) -> (-118.2831, 1038.7555)
  line L436 (-118.2831, 1038.7555) -> (-146.9619, 997.7979)
  line L437 (-200.2068, 1035.0804) -> (-241.1644, 1063.7592)
  line L438 (-241.1644, 1063.7592) -> (-212.4856, 1104.7168)
  line L439 (-212.4856, 1104.7168) -> (-171.528, 1076.038)
  line L440 (-171.528, 1076.038) -> (-200.2068, 1035.0804)
  line L441 (-253.4517, 1072.3628) -> (-294.4093, 1101.0417)
  line L442 (-294.4093, 1101.0417) -> (-265.7305, 1141.9993)
  line L443 (-265.7305, 1141.9993) -> (-224.7729, 1113.3204)
  line L444 (-224.7729, 1113.3204) -> (-253.4517, 1072.3628)
  line L445 (-306.6966, 1109.6453) -> (-347.6542, 1138.3241)
  line L446 (-347.6542, 1138.3241) -> (-318.9754, 1179.2817)
  line L447 (-318.9754, 1179.2817) -> (-278.0178, 1150.6029)
  line L448 (-278.0178, 1150.6029) -> (-306.6966, 1109.6453)
  line L449 (-359.9415, 1146.9278) -> (-400.8991, 1175.6066)
  line L450 (-400.8991, 1175.6066) -> (-372.2202, 1216.5642)
  line L451 (-372.2202, 1216.5642) -> (-331.2626, 1187.8854)
  line L452 (-331.2626, 1187.8854) -> (-359.9415, 1146.9278)
  line L453 (-413.1863, 1184.2102) -> (-454.1439, 1212.8891)
  line L454 (-454.1439, 1212.8891) -> (-425.4651, 1253.8467)
  line L455 (-425.4651, 1253.8467) -> (-384.5075, 1225.1678)
  line L456 (-384.5075, 1225.1678) -> (-413.1863, 1184.2102)
  line L457 (-466.4312, 1221.4927) -> (-507.3888, 1250.1715)
  line L458 (-507.3888, 1250.1715) -> (-478.71, 1291.1291)
  line L459 (-478.71, 1291.1291) -> (-437.7524, 1262.4503)
  line L460 (-437.7524, 1262.4503) -> (-466.4312, 1221.4927)
  line L461 (-519.6761, 1258.7752) -> (-560.6337, 1287.454)
  line L462 (-560.6337, 1287.454) -> (-531.9549, 1328.4116)
  line L463 (-531.9549, 1328.4116) -> (-490.9973, 1299.7328)
  line L464 (-490.9973, 1299.7328) -> (-519.6761, 1258.7752)
  line L465 (-572.921, 1296.0576) -> (-613.8786, 1324.7365)
  line L466 (-613.8786, 1324.7365) -> (-585.1998, 1365.6941)
  line L467 (-585.1998, 1365.6941) -> (-544.2422, 1337.0152)
  line L468 (-544.2422, 1337.0152) -> (-572.921, 1296.0576)
  line L469 (-626.1659, 1333.3401) -> (-667.1235, 1362.0189)
  line L470 (-667.1235, 1362.0189) -> (-638.4447, 1402.9765)
  line L471 (-638.4447, 1402.9765) -> (-597.4871, 1374.2977)
  line L472 (-597.4871, 1374.2977) -> (-626.1659, 1333.3401)
  line L473 (-679.4108, 1370.6226) -> (-720.3684, 1399.3014)
  line L474 (-720.3684, 1399.3014) -> (-691.6895, 1440.259)
  line L475 (-691.6895, 1440.259) -> (-650.7319, 1411.5802)
  line L476 (-650.7319, 1411.5802) -> (-679.4108, 1370.6226)
  line L477 (-732.6556, 1407.905) -> (-773.6132, 1436.5839)
  line L478 (-773.6132, 1436.5839) -> (-744.9344, 1477.5415)
  line L479 (-744.9344, 1477.5415) -> (-703.9768, 1448.8626)
  line L480 (-703.9768, 1448.8626) -> (-732.6556, 1407.905)
  line L481 (-24.5097, 832.7056) -> (-65.4673, 861.3844)
  line L482 (-65.4673, 861.3844) -> (-36.7885, 902.342)
  line L483 (-36.7885, 902.342) -> (4.1691, 873.6632)
  line L484 (4.1691, 873.6632) -> (-24.5097, 832.7056)
  line L485 (-77.7546, 869.9881) -> (-118.7122, 898.6669)
  line L486 (-118.7122, 898.6669) -> (-90.0334, 939.6245)
  line L487 (-90.0334, 939.6245) -> (-49.0758, 910.9457)
  line L488 (-49.0758, 910.9457) -> (-77.7546, 869.9881)
  line L489 (-130.9995, 907.2705) -> (-171.9571, 935.9494)
  line L490 (-171.9571, 935.9494) -> (-143.2783, 976.907)
  line L491 (-143.2783, 976.907) -> (-102.3207, 948.2281)
  line L492 (-102.3207, 948.2281) -> (-130.9995, 907.2705)
  line L493 (-184.2444, 944.553) -> (-225.202, 973.2318)
  line L494 (-225.202, 973.2318) -> (-196.5232, 1014.1894)
  line L495 (-196.5232, 1014.1894) -> (-155.5656, 985.5106)
  line L496 (-155.5656, 985.5106) -> (-184.2444, 944.553)
  line L497 (-237.4893, 981.8355) -> (-278.4469, 1010.5143)
  line L498 (-278.4469, 1010.5143) -> (-249.7681, 1051.4719)
  line L499 (-249.7681, 1051.4719) -> (-208.8105, 1022.7931)
  line L500 (-208.8105, 1022.7931) -> (-237.4893, 981.8355)
  line L501 (-290.7342, 1019.1179) -> (-331.6918, 1047.7968)
  line L502 (-331.6918, 1047.7968) -> (-303.0129, 1088.7544)
  line L503 (-303.0129, 1088.7544) -> (-262.0553, 1060.0755)
  line L504 (-262.0553, 1060.0755) -> (-290.7342, 1019.1179)
  line L505 (-343.979, 1056.4004) -> (-384.9366, 1085.0792)
  line L506 (-384.9366, 1085.0792) -> (-356.2578, 1126.0368)
  line L507 (-356.2578, 1126.0368) -> (-315.3002, 1097.358)
  line L508 (-315.3002, 1097.358) -> (-343.979, 1056.4004)
  line L509 (-397.2239, 1093.6829) -> (-438.1815, 1122.3617)
  line L510 (-438.1815, 1122.3617) -> (-409.5027, 1163.3193)
  line L511 (-409.5027, 1163.3193) -> (-368.5451, 1134.6405)
  line L512 (-368.5451, 1134.6405) -> (-397.2239, 1093.6829)
  line L513 (-450.4688, 1130.9654) -> (-491.4264, 1159.6442)
  line L514 (-491.4264, 1159.6442) -> (-462.7476, 1200.6018)
  line L515 (-462.7476, 1200.6018) -> (-421.79, 1171.923)
  line L516 (-421.79, 1171.923) -> (-450.4688, 1130.9654)
  line L517 (-503.7137, 1168.2478) -> (-544.6713, 1196.9266)
  line L518 (-544.6713, 1196.9266) -> (-515.9925, 1237.8842)
  line L519 (-515.9925, 1237.8842) -> (-475.0349, 1209.2054)
  line L520 (-475.0349, 1209.2054) -> (-503.7137, 1168.2478)
  line L521 (-556.9586, 1205.5303) -> (-597.9162, 1234.2091)
  line L522 (-597.9162, 1234.2091) -> (-569.2374, 1275.1667)
  line L523 (-569.2374, 1275.1667) -> (-528.2798, 1246.4879)
  line L524 (-528.2798, 1246.4879) -> (-556.9586, 1205.5303)
  line L525 (-610.2035, 1242.8128) -> (-651.1611, 1271.4916)
  line L526 (-651.1611, 1271.4916) -> (-622.4822, 1312.4492)
  line L527 (-622.4822, 1312.4492) -> (-581.5246, 1283.7704)
  line L528 (-581.5246, 1283.7704) -> (-610.2035, 1242.8128)
  line L529 (-663.4483, 1280.0952) -> (-704.4059, 1308.774)
  line L530 (-704.4059, 1308.774) -> (-675.7271, 1349.7316)
  line L531 (-675.7271, 1349.7316) -> (-634.7695, 1321.0528)
  line L532 (-634.7695, 1321.0528) -> (-663.4483, 1280.0952)
  line L533 (-716.6932, 1317.3777) -> (-757.6508, 1346.0565)
  line L534 (-757.6508, 1346.0565) -> (-728.972, 1387.0141)
  line L535 (-728.972, 1387.0141) -> (-688.0144, 1358.3353)
  line L536 (-688.0144, 1358.3353) -> (-716.6932, 1317.3777)
  line L537 (-769.9381, 1354.6602) -> (-810.8957, 1383.339)
  line L538 (-810.8957, 1383.339) -> (-782.2169, 1424.2966)
  line L539 (-782.2169, 1424.2966) -> (-741.2593, 1395.6178)
  line L540 (-741.2593, 1395.6178) -> (-769.9381, 1354.6602)
  line L541 (-61.7922, 779.4607) -> (-102.7498, 808.1395)
  line L542 (-102.7498, 808.1395) -> (-74.071, 849.0971)
  line L543 (-74.071, 849.0971) -> (-33.1134, 820.4183)
  line L544 (-33.1134, 820.4183) -> (-61.7922, 779.4607)
  line L545 (-115.0371, 816.7432) -> (-155.9947, 845.422)
  line L546 (-155.9947, 845.422) -> (-127.3159, 886.3796)
  line L547 (-127.3159, 886.3796) -> (-86.3583, 857.7008)
  line L548 (-86.3583, 857.7008) -> (-115.0371, 816.7432)
  line L549 (-168.282, 854.0257) -> (-209.2396, 882.7045)
  line L550 (-209.2396, 882.7045) -> (-180.5608, 923.6621)
  line L551 (-180.5608, 923.6621) -> (-139.6032, 894.9833)
  line L552 (-139.6032, 894.9833) -> (-168.282, 854.0257)
  line L553 (-221.5269, 891.3081) -> (-262.4845, 919.9869)
  line L554 (-262.4845, 919.9869) -> (-233.8056, 960.9446)
  line L555 (-233.8056, 960.9446) -> (-192.848, 932.2657)
  line L556 (-192.848, 932.2657) -> (-221.5269, 891.3081)
  line L557 (-274.7717, 928.5906) -> (-315.7293, 957.2694)
  line L558 (-315.7293, 957.2694) -> (-287.0505, 998.227)
  line L559 (-287.0505, 998.227) -> (-246.0929, 969.5482)
  line L560 (-246.0929, 969.5482) -> (-274.7717, 928.5906)
  line L561 (-328.0166, 965.8731) -> (-368.9742, 994.5519)
  line L562 (-368.9742, 994.5519) -> (-340.2954, 1035.5095)
  line L563 (-340.2954, 1035.5095) -> (-299.3378, 1006.8307)
  line L564 (-299.3378, 1006.8307) -> (-328.0166, 965.8731)
  line L565 (-381.2615, 1003.1555) -> (-422.2191, 1031.8344)
  line L566 (-422.2191, 1031.8344) -> (-393.5403, 1072.792)
  line L567 (-393.5403, 1072.792) -> (-352.5827, 1044.1131)
  line L568 (-352.5827, 1044.1131) -> (-381.2615, 1003.1555)
  line L569 (-434.5064, 1040.438) -> (-475.464, 1069.1168)
  line L570 (-475.464, 1069.1168) -> (-446.7852, 1110.0744)
  line L571 (-446.7852, 1110.0744) -> (-405.8276, 1081.3956)
  line L572 (-405.8276, 1081.3956) -> (-434.5064, 1040.438)
  line L573 (-487.7513, 1077.7205) -> (-528.7089, 1106.3993)
  line L574 (-528.7089, 1106.3993) -> (-500.0301, 1147.3569)
  line L575 (-500.0301, 1147.3569) -> (-459.0725, 1118.6781)
  line L576 (-459.0725, 1118.6781) -> (-487.7513, 1077.7205)
  line L577 (-540.9962, 1115.0029) -> (-581.9538, 1143.6818)
  line L578 (-581.9538, 1143.6818) -> (-553.2749, 1184.6394)
  line L579 (-553.2749, 1184.6394) -> (-512.3173, 1155.9605)
  line L580 (-512.3173, 1155.9605) -> (-540.9962, 1115.0029)
  line L581 (-594.241, 1152.2854) -> (-635.1986, 1180.9642)
  line L582 (-635.1986, 1180.9642) -> (-606.5198, 1221.9218)
  line L583 (-606.5198, 1221.9218) -> (-565.5622, 1193.243)
  line L584 (-565.5622, 1193.243) -> (-594.241, 1152.2854)
  line L585 (-647.4859, 1189.5679) -> (-688.4435, 1218.2467)
  line L586 (-688.4435, 1218.2467) -> (-659.7647, 1259.2043)
  line L587 (-659.7647, 1259.2043) -> (-618.8071, 1230.5255)
  line L588 (-618.8071, 1230.5255) -> (-647.4859, 1189.5679)
  line L589 (-700.7308, 1226.8503) -> (-741.6884, 1255.5292)
  line L590 (-741.6884, 1255.5292) -> (-713.0096, 1296.4868)
  line L591 (-713.0096, 1296.4868) -> (-672.052, 1267.8079)
  line L592 (-672.052, 1267.8079) -> (-700.7308, 1226.8503)
  line L593 (-753.9757, 1264.1328) -> (-794.9333, 1292.8116)
  line L594 (-794.9333, 1292.8116) -> (-766.2545, 1333.7692)
  line L595 (-766.2545, 1333.7692) -> (-725.2969, 1305.0904)
  line L596 (-725.2969, 1305.0904) -> (-753.9757, 1264.1328)
  line L597 (-807.2206, 1301.4153) -> (-848.1782, 1330.0941)
  line L598 (-848.1782, 1330.0941) -> (-819.4994, 1371.0517)
  line L599 (-819.4994, 1371.0517) -> (-778.5418, 1342.3729)
  line L600 (-778.5418, 1342.3729) -> (-807.2206, 1301.4153)
  line L601 (-99.0747, 726.2158) -> (-140.0323, 754.8947)
  line L602 (-140.0323, 754.8947) -> (-111.3535, 795.8523)
  line L603 (-111.3535, 795.8523) -> (-70.3959, 767.1734)
  line L604 (-70.3959, 767.1734) -> (-99.0747, 726.2158)
  line L605 (-152.3196, 763.4983) -> (-193.2772, 792.1771)
  line L606 (-193.2772, 792.1771) -> (-164.5983, 833.1347)
  line L607 (-164.5983, 833.1347) -> (-123.6407, 804.4559)
  line L608 (-123.6407, 804.4559) -> (-152.3196, 763.4983)
  line L609 (-205.5644, 800.7808) -> (-246.5221, 829.4596)
  line L610 (-246.5221, 829.4596) -> (-217.8432, 870.4172)
  line L611 (-217.8432, 870.4172) -> (-176.8856, 841.7384)
  line L612 (-176.8856, 841.7384) -> (-205.5644, 800.7808)
  line L613 (-258.8093, 838.0632) -> (-299.7669, 866.7421)
  line L614 (-299.7669, 866.7421) -> (-271.0881, 907.6997)
  line L615 (-271.0881, 907.6997) -> (-230.1305, 879.0208)
  line L616 (-230.1305, 879.0208) -> (-258.8093, 838.0632)
  line L617 (-312.0542, 875.3457) -> (-353.0118, 904.0245)
  line L618 (-353.0118, 904.0245) -> (-324.333, 944.9821)
  line L619 (-324.333, 944.9821) -> (-283.3754, 916.3033)
  line L620 (-283.3754, 916.3033) -> (-312.0542, 875.3457)
  line L621 (-365.2991, 912.6282) -> (-406.2567, 941.307)
  line L622 (-406.2567, 941.307) -> (-377.5779, 982.2646)
  line L623 (-377.5779, 982.2646) -> (-336.6203, 953.5858)
  line L624 (-336.6203, 953.5858) -> (-365.2991, 912.6282)
  line L625 (-418.544, 949.9106) -> (-459.5016, 978.5895)
  line L626 (-459.5016, 978.5895) -> (-430.8228, 1019.5471)
  line L627 (-430.8228, 1019.5471) -> (-389.8652, 990.8683)
  line L628 (-389.8652, 990.8683) -> (-418.544, 949.9106)
  line L629 (-471.7889, 987.1931) -> (-512.7465, 1015.8719)
  line L630 (-512.7465, 1015.8719) -> (-484.0676, 1056.8295)
  line L631 (-484.0676, 1056.8295) -> (-443.11, 1028.1507)
  line L632 (-443.11, 1028.1507) -> (-471.7889, 987.1931)
  line L633 (-525.0337, 1024.4756) -> (-565.9913, 1053.1544)
  line L634 (-565.9913, 1053.1544) -> (-537.3125, 1094.112)
  line L635 (-537.3125, 1094.112) -> (-496.3549, 1065.4332)
  line L636 (-496.3549, 1065.4332) -> (-525.0337, 1024.4756)
  line L637 (-578.2786, 1061.7581) -> (-619.2362, 1090.4369)
  line L638 (-619.2362, 1090.4369) -> (-590.5574, 1131.3945)
  line L639 (-590.5574, 1131.3945) -> (-549.5998, 1102.7157)
  line L640 (-549.5998, 1102.7157) -> (-578.2786, 1061.7581)
  line L641 (-631.5235, 1099.0405) -> (-672.4811, 1127.7193)
  line L642 (-672.4811, 1127.7193) -> (-643.8023, 1168.6769)
  line L643 (-643.8023, 1168.6769) -> (-602.8447, 1139.9981)
  line L644 (-602.8447, 1139.9981) -> (-631.5235, 1099.0405)
  line L645 (-684.7684, 1136.323) -> (-725.726, 1165.0018)
  line L646 (-725.726, 1165.0018) -> (-697.0472, 1205.9594)
  line L647 (-697.0472, 1205.9594) -> (-656.0896, 1177.2806)
  line L648 (-656.0896, 1177.2806) -> (-684.7684, 1136.323)
  line L649 (-738.0133, 1173.6055) -> (-778.9709, 1202.2843)
  line L650 (-778.9709, 1202.2843) -> (-750.2921, 1243.2419)
  line L651 (-750.2921, 1243.2419) -> (-709.3345, 1214.5631)
  line L652 (-709.3345, 1214.5631) -> (-738.0133, 1173.6055)
  line L653 (-791.2582, 1210.8879) -> (-832.2158, 1239.5667)
  line L654 (-832.2158, 1239.5667) -> (-803.5369, 1280.5244)
  line L655 (-803.5369, 1280.5244) -> (-762.5793, 1251.8455)
  line L656 (-762.5793, 1251.8455) -> (-791.2582, 1210.8879)
  line L657 (-844.503, 1248.1704) -> (-885.4606, 1276.8492)
  line L658 (-885.4606, 1276.8492) -> (-856.7818, 1317.8068)
  line L659 (-856.7818, 1317.8068) -> (-815.8242, 1289.128)
  line L660 (-815.8242, 1289.128) -> (-844.503, 1248.1704)
  line L661 (-136.3572, 672.971) -> (-177.3148, 701.6498)
  line L662 (-177.3148, 701.6498) -> (-148.6359, 742.6074)
  line L663 (-148.6359, 742.6074) -> (-107.6783, 713.9286)
  line L664 (-107.6783, 713.9286) -> (-136.3572, 672.971)
  line L665 (-189.602, 710.2534) -> (-230.5596, 738.9322)
  line L666 (-230.5596, 738.9322) -> (-201.8808, 779.8898)
  line L667 (-201.8808, 779.8898) -> (-160.9232, 751.211)
  line L668 (-160.9232, 751.211) -> (-189.602, 710.2534)
  line L669 (-242.8469, 747.5359) -> (-283.8045, 776.2147)
  line L670 (-283.8045, 776.2147) -> (-255.1257, 817.1723)
  line L671 (-255.1257, 817.1723) -> (-214.1681, 788.4935)
  line L672 (-214.1681, 788.4935) -> (-242.8469, 747.5359)
  line L673 (-296.0918, 784.8184) -> (-337.0494, 813.4972)
  line L674 (-337.0494, 813.4972) -> (-308.3706, 854.4548)
  line L675 (-308.3706, 854.4548) -> (-267.413, 825.776)
  line L676 (-267.413, 825.776) -> (-296.0918, 784.8184)
  line L677 (-349.3367, 822.1008) -> (-390.2943, 850.7797)
  line L678 (-390.2943, 850.7797) -> (-361.6155, 891.7373)
  line L679 (-361.6155, 891.7373) -> (-320.6579, 863.0584)
  line L680 (-320.6579, 863.0584) -> (-349.3367, 822.1008)
  line L681 (-402.5816, 859.3833) -> (-443.5392, 888.0621)
  line L682 (-443.5392, 888.0621) -> (-414.8603, 929.0197)
  line L683 (-414.8603, 929.0197) -> (-373.9027, 900.3409)
  line L684 (-373.9027, 900.3409) -> (-402.5816, 859.3833)
  line L685 (-455.8264, 896.6658) -> (-496.7841, 925.3446)
  line L686 (-496.7841, 925.3446) -> (-468.1052, 966.3022)
  line L687 (-468.1052, 966.3022) -> (-427.1476, 937.6234)
  line L688 (-427.1476, 937.6234) -> (-455.8264, 896.6658)
  line L689 (-509.0713, 933.9482) -> (-550.0289, 962.6271)
  line L690 (-550.0289, 962.6271) -> (-521.3501, 1003.5847)
  line L691 (-521.3501, 1003.5847) -> (-480.3925, 974.9058)
  line L692 (-480.3925, 974.9058) -> (-509.0713, 933.9482)
  line L693 (-562.3162, 971.2307) -> (-603.2738, 999.9095)
  line L694 (-603.2738, 999.9095) -> (-574.595, 1040.8671)
  line L695 (-574.595, 1040.8671) -> (-533.6374, 1012.1883)
  line L696 (-533.6374, 1012.1883) -> (-562.3162, 971.2307)
  line L697 (-615.5611, 1008.5132) -> (-656.5187, 1037.192)
  line L698 (-656.5187, 1037.192) -> (-627.8399, 1078.1496)
  line L699 (-627.8399, 1078.1496) -> (-586.8823, 1049.4708)
  line L700 (-586.8823, 1049.4708) -> (-615.5611, 1008.5132)
  line L701 (-668.806, 1045.7956) -> (-709.7636, 1074.4745)
  line L702 (-709.7636, 1074.4745) -> (-681.0848, 1115.4321)
  line L703 (-681.0848, 1115.4321) -> (-640.1272, 1086.7532)
  line L704 (-640.1272, 1086.7532) -> (-668.806, 1045.7956)
  line L705 (-722.0509, 1083.0781) -> (-763.0085, 1111.7569)
  line L706 (-763.0085, 1111.7569) -> (-734.3296, 1152.7145)
  line L707 (-734.3296, 1152.7145) -> (-693.372, 1124.0357)
  line L708 (-693.372, 1124.0357) -> (-722.0509, 1083.0781)
  line L709 (-775.2957, 1120.3606) -> (-816.2533, 1149.0394)
  line L710 (-816.2533, 1149.0394) -> (-787.5745, 1189.997)
  line L711 (-787.5745, 1189.997) -> (-746.6169, 1161.3182)
  line L712 (-746.6169, 1161.3182) -> (-775.2957, 1120.3606)
  line L713 (-828.5406, 1157.643) -> (-869.4982, 1186.3219)
  line L714 (-869.4982, 1186.3219) -> (-840.8194, 1227.2795)
  line L715 (-840.8194, 1227.2795) -> (-799.8618, 1198.6006)
  line L716 (-799.8618, 1198.6006) -> (-828.5406, 1157.643)
  line L717 (-881.7855, 1194.9255) -> (-922.7431, 1223.6043)
  line L718 (-922.7431, 1223.6043) -> (-894.0643, 1264.5619)
  line L719 (-894.0643, 1264.5619) -> (-853.1067, 1235.8831)
  line L720 (-853.1067, 1235.8831) -> (-881.7855, 1194.9255)
  line L721 (-173.6396, 619.7261) -> (-214.5972, 648.4049)
  line L722 (-214.5972, 648.4049) -> (-185.9184, 689.3625)
  line L723 (-185.9184, 689.3625) -> (-144.9608, 660.6837)
  line L724 (-144.9608, 660.6837) -> (-173.6396, 619.7261)
  line L725 (-226.8845, 657.0085) -> (-267.8421, 685.6874)
  line L726 (-267.8421, 685.6874) -> (-239.1633, 726.645)
  line L727 (-239.1633, 726.645) -> (-198.2057, 697.9661)
  line L728 (-198.2057, 697.9661) -> (-226.8845, 657.0085)
  line L729 (-280.1294, 694.291) -> (-321.087, 722.9698)
  line L730 (-321.087, 722.9698) -> (-292.4082, 763.9274)
  line L731 (-292.4082, 763.9274) -> (-251.4506, 735.2486)
  line L732 (-251.4506, 735.2486) -> (-280.1294, 694.291)
  line L733 (-333.3743, 731.5735) -> (-374.3319, 760.2523)
  line L734 (-374.3319, 760.2523) -> (-345.653, 801.2099)
  line L735 (-345.653, 801.2099) -> (-304.6954, 772.5311)
  line L736 (-304.6954, 772.5311) -> (-333.3743, 731.5735)
  line L737 (-386.6192, 768.8559) -> (-427.5768, 797.5348)
  line L738 (-427.5768, 797.5348) -> (-398.8979, 838.4924)
  line L739 (-398.8979, 838.4924) -> (-357.9403, 809.8135)
  line L740 (-357.9403, 809.8135) -> (-386.6192, 768.8559)
  line L741 (-439.864, 806.1384) -> (-480.8216, 834.8172)
  line L742 (-480.8216, 834.8172) -> (-452.1428, 875.7748)
  line L743 (-452.1428, 875.7748) -> (-411.1852, 847.096)
  line L744 (-411.1852, 847.096) -> (-439.864, 806.1384)
  line L745 (-493.1089, 843.4209) -> (-534.0665, 872.0997)
  line L746 (-534.0665, 872.0997) -> (-505.3877, 913.0573)
  line L747 (-505.3877, 913.0573) -> (-464.4301, 884.3785)
  line L748 (-464.4301, 884.3785) -> (-493.1089, 843.4209)
  line L749 (-546.3538, 880.7034) -> (-587.3114, 909.3822)
  line L750 (-587.3114, 909.3822) -> (-558.6326, 950.3398)
  line L751 (-558.6326, 950.3398) -> (-517.675, 921.661)
  line L752 (-517.675, 921.661) -> (-546.3538, 880.7034)
  line L753 (-599.5987, 917.9858) -> (-640.5563, 946.6646)
  line L754 (-640.5563, 946.6646) -> (-611.8775, 987.6222)
  line L755 (-611.8775, 987.6222) -> (-570.9199, 958.9434)